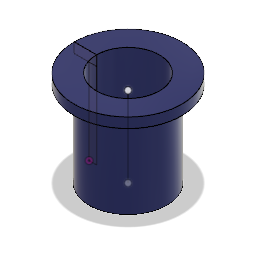
Adaptateur feutre (Autodesk Fusion 360 design; units mm, degrees)
Autodesk Fusion 360 part; units mm, degrees
sketch "Sketch tranche" plane through (0, 0, 0) normal (0, 0, 1) x (1, 0, 0)
  line L0 (0, 0) -> (1.5, 0)
  line L1 (1.5, 0) -> (1.5, 17)
  line L2 (1.5, 17) -> (0, 17)
  line L3 (0, 17) -> (0, 0)
  line L4 (7.75, 0) -> (7.75, 16)
  line L5 (1.5, 17) -> (-3, 17)
  line L6 (-3, 17) -> (-3, 19)
  line L7 (-3, 19) -> (1.5, 19)
  line L8 (1.5, 19) -> (1.5, 17)
  dimension "d1" = 1.5
  dimension "d2" = 17
  dimension "d3" = 7.75
  dimension "d4" = 3
  dimension "d5" = 2
  constraint horizontal L0
  constraint vertical L1
  constraint horizontal L2
  constraint vertical L3
  constraint coincident L0.start L3.end
  constraint perpendicular L2 L4
  constraint horizontal L5
  constraint vertical L6
  constraint horizontal L7
  constraint vertical L8
  measures "d1" distance of L1 L3
  measures "d2" distance of L0 L2
  measures "d3" distance of L3 L4
  measures "d4" distance of L3 L6
  measures "d5" distance of L5 L7
revolve "Revolution tranche" add sketch "Sketch tranche" angle 360 about axis through (7.75, 0, 0) along (0, 1, 0)
named bodies: "Adaptateur feutre"
